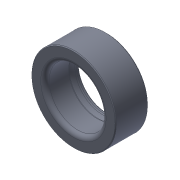
# Autodesk Inventor part: NA-45-h-Crown-127
Saved by Autodesk Inventor 2020.3 (Build 243373010, 373A)
## iProperties
Created: 2020-09-21
Part Number: NA-45-h-Crown-127
Material: 19 436.4
Description: STAHOVACI KROUZEK
Document SubType Name: Modeling
Designer: Jurek
Density: 7.85 g/cm^3
Appearance: RAL 7040 Window Grey(1)
Mass: 284.972 g
Surface Area: 102.095 cm^2
Volume: 36.3022 cm^3
User Status: Rozpracováno
Category: B
Hmotnost (kg): 0,28
Rozmer_A: 60
Rozmer_B: 23,5
Rozmer_C: 0
Rozmer_D: 23,5
Rada vyrobku: 4100
Prumer nadobky: 45
Cislo artiklu: 4451101284
Jednotka: ks
Cisty rozmer: =Ø<Rozmer_A> - <Rozmer_D>
Predpona: Ø
Stroj na lince: Stahovací lis
RAZ Poznamka 1: ISO 2768-mH
RAZ Poznamka 2: NEOZNAČENÉ HRANY OJEHLIT
RAZ Poznamka 3: KALIT NA 58 - 60 HRc
DXF: Ne
QAD_code: M
Rizeni davek: L
Author: Správce
Revision Number: 00
Autodesk Inventor part; units mm, degrees
ref_plane "YZ Plane" through (0, 0, 0) normal (1, 0, 0) x (0, 1, 0)
ref_plane "XZ Plane" through (0, 0, 0) normal (0, 1, 0) x (-1, 0, 0)
ref_plane "XY Plane" through (0, 0, 0) normal (0, 0, 1) x (1, 0, 0)
sketch "Náčrt1" plane through (0, 0, 0) normal (0, 0, 1) x (1, 0, 0)
  line L0 (0, 0) -> (0, 63.6053)
  line L1 (20.025, 23.5) -> (30, 23.5)
  line L2 (30, 23.5) -> (30, 0)
  line L3 (30, 0) -> (23.2, 0)
  arc A0 (20.2, 16.8138) -> (20.1389, 17.2376) centre (18.7, 16.8138) ccw
  arc A1 (19.65, 20.6279) -> (20.1389, 17.2376) centre (31.65, 20.6279) ccw
  arc A2 (20.2, 3) -> (23.2, 0) centre (23.2, 3) ccw
  line L4 (20.2, 16.8138) -> (20.2, 3)
  arc A3 (20.1, 16.9) -> (19.65, 18.2) centre (18.6153, 17.114) ccw construction
  arc A4 (19.2447, 18.8659) -> (19.65, 18.2) centre (20.6847, 19.286) ccw construction
  arc A5 (19.2447, 18.8659) -> (18.8277, 19.5429) centre (17.8047, 18.4458) ccw construction
  line L5 (13.5384, 24.4753) -> (18.8277, 19.5429) construction
  arc A6 (18.8277, 19.5429) -> (13.5384, 24.4753) centre (7.4354, 12.6284) ccw construction
  arc A7 (20.025, 23.5) -> (19.725, 23.2) centre (20.025, 23.2) ccw
  line L6 (19.65, 21.8279) -> (19.65, 20.6279)
  line L7 (19.65, 21.8279) -> (19.725, 23.0541)
  line L8 (19.65, 21.8279) -> (20.8785, 21.8279) construction
  line L9 (19.725, 23.2) -> (19.725, 23.0541)
  point P0 (19.7148, 23.5)
  dimension "d0" = 60
  dimension "d1" = 40.4
  dimension "d3" = 23.5
  dimension "d8" = 1.5
  dimension "d9" = 12
  dimension "d11" = 3
  dimension "d13" = 21.8279
  dimension "d30" = 16.8138
  dimension "d39" = 0.5
  dimension "d41" = 0.3
  dimension "d43" = 1.2
  dimension "d44" = 39.3
  dimension "d45" = 86.5
  dimension "d46" = 39.45
  constraints: 20 end point, 15 point on circle, 7 centre point, 6 point on line, 6 tangent, 3 vertical, 2 perpendicular, 1 equal length, 1 horizontal, 1 parallel, 19 other
  measures "d0" diameter of L2 L0
  measures "d1" diameter of L4.start L0
  measures "d3" distance between parallel lines of L3 L1
  measures "d8" radius of A0
  measures "d9" radius of A1
  measures "d11" radius of A2
  measures "d13" distance from line of L6.start L3
  measures "d30" distance from line of L4.start L3
  measures "d39" distance edge to line of A6 L5
  measures "d41" radius of A7
  measures "d43" distance of L6.end L6.start
  measures "d44" diameter of L6 L0
  measures "d45" angle of L8 L7
  measures "d46" diameter of L9 L0
revolve "Rotace1" add sketch "Náčrt1" angle 360 about axis through (0, 0, 0) along (0, 1, 0)
chamfer "Zkosení1" distance 0.5 angle 45 1 edges at (-30, 0, 0)
chamfer "Zkosení3" distance 1 angle 45 1 edges at (-30, 23.5, 0)
equation "\"Rozmer_B\" = 23.5"
equation "\"Rozmer_C\" = 0"
equation "\"Rozmer_D\" = 23.5"
